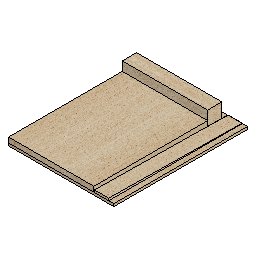
model (Autodesk Fusion 360 design; units mm, degrees)
Autodesk Fusion 360 part; units mm, degrees
sketch "Sketch1" plane through (0, 0, 0) normal (0, 0, 1) x (1, 0, 0)
  line L0 (0, 0) -> (300, 0)
  line L1 (300, 0) -> (300, 400)
  line L2 (300, 400) -> (0, 400)
  line L3 (0, 400) -> (0, 0)
  line L4 (0, 400) -> (0, 470)
  line L5 (0, 470) -> (370, 470)
  line L6 (370, 470) -> (370, 0)
  line L7 (370, 0) -> (300, 0)
  line L8 (0, 450) -> (300, 450)
  line L9 (300, 450) -> (300, 400)
  line L10 (302, 470) -> (302, 0)
  line L11 (352, 0) -> (352, 470)
  dimension "d1" = 400
  dimension "d2" = 300
  dimension "d3" = 70
  dimension "d4" = 70
  dimension "d5" = 50
  dimension "d6" = 50
  dimension "d7" = 2
  constraint horizontal L0
  constraint vertical L1
  constraint horizontal L2
  constraint vertical L3
  constraint coincident L0.start L3.end
  constraint horizontal L7
  constraint vertical L6
  constraint horizontal L5
  constraint vertical L4
  constraint coincident L4 L8.start
  constraint vertical L9
  constraint horizontal L8
  constraint coincident L5 L10.start
  constraint coincident L7 L10.end
  constraint coincident L7 L11.start
  constraint coincident L5 L11.end
  constraint vertical L10
  constraint vertical L11
  measures "d1" distance of L0.start L2.end
  measures "d2" distance of L0.start L0.end
  measures "d3" distance of L2.end L4.end
  measures "d4" distance of L1 L6
  measures "d5" distance of L2 L8
  measures "d6" distance of L10 L11
  measures "d7" distance of L1 L10
extrude "Extrude1" add sketch "Sketch1" against normal blind 9 makes body 1
extrude "Extrude2" add sketch "Sketch1" along normal blind 18 separate body contours L0 L1 L2 L3 makes body 2
extrude "Extrude3" add sketch "Sketch1" along normal blind 50 separate body contours L2 L4 L8 L9 makes body 3
extrude "Extrude4" add sketch "Sketch1" along normal blind 8 separate body contours L5 L7 L10 L11 makes body 4
draft "Draft1" angle -0.8 neutral plane through (352, 0, 0) pull (0, -1, 0) 1 faces at (318.6667, 313.3333, 8) on bodies 4
